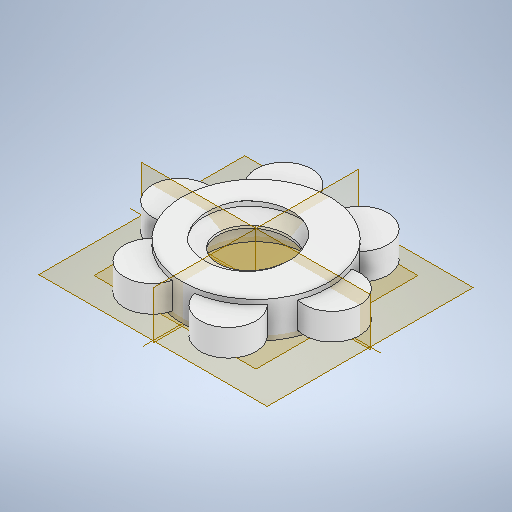
# Autodesk Inventor part: bearing-clamp
Saved by Autodesk Inventor 2025.2 (Build 292293000, 293)
## iProperties
Created: 2024-12-19
Part Number: bearing-clamp
Material: PC/ABS Plastic
Document SubType Name: Modeling
Designer: yehorderehus
Density: 1.1 g/cm^3
Appearance: Smooth - White
Mass: 0.72271 g
Surface Area: 7.25269 cm^2
Volume: 0.657009 cm^3
Author: yehorderehus
Autodesk Inventor part; units mm, degrees
sketch "Sketch1" plane through (0, 0, 0) normal (0, 1, 0) x (-1, 0, 0)
  circle A0 centre (0, 0) radius 6.1
  circle A1 centre (0, 0) radius 4
  dimension "d0" = 12.2
  dimension "d1" = 8
  constraints: 2 centre point, 2 coincident
  measures "d0" diameter of A0
  measures "d1" diameter of A1
extrude "Extrusion1" add sketch "Sketch1" along normal blind 3
ref_plane "Work Plane1" through (0, 0.4, 0) normal (0, 1, 0) x (-1, 0, 0)
sketch "Sketch2" plane through (0, 0.4, 0) normal (0, 1, 0) x (-1, 0, 0)
  circle A0 centre (0, 0) radius 8.6 construction
  circle A1 centre (-6.3, 0) radius 2.3
  circle A2 centre (0, 0) radius 4 projected
  dimension "d5" = 17.2
  constraints: 2 centre point, 2 tangent, 1 coincident
  measures "d5" diameter of A0
extrude "Extrusion2" add sketch "Sketch2" along normal blind 2.2 contours A1
pattern_circular "Circular Pattern1" count 6 over 360 about axis through (0, -10, 0) along (0, 1, 0) of "Extrusion2"
sketch "Sketch3" plane through (0, 0, 0) normal (1, 0, 0) x (0, 1, 0)
  line L0 (3, 4) -> (0, 4) projected
  line L1 (0, 4) -> (0.6, 2.9)
  line L2 (0, -6.1) -> (0, 6.1) projected
  line L3 (0, 8.54) -> (0, -8.54) projected
  line L4 (0.6, 2.9) -> (0.8, 2.9)
  line L5 (0.8, 2.9) -> (1.4, 4)
  line L6 (1.4, 4) -> (0, 4)
  point P0 (0, 0)
  dimension "d12" = 0.2
  dimension "d13" = 1.1
  dimension "d14" = 1.4
  constraints: 8 end point, 3 point on line, 1 collinear, 1 equal length, 1 horizontal
  measures "d12" distance of L1.end L4.end
  measures "d13" distance between parallel lines of L0 L4
  measures "d14" distance of L5.end L0.end
coil "Coil1" sketch "Sketch3" operation add axis through (0, -10, 0) along (0, 1, 0) pitch 1.8 turns 2.4 hand right
sketch "Sketch4" plane through (0, 3, 0) normal (0, 1, 0) x (1, 0, 0)
  circle A0 centre (0, 0) radius 6.1
  constraints: 1 centre point, 1 coincident
extrude "Extrusion3" cut sketch "Sketch4" along normal blind 10
body "Solid1"
